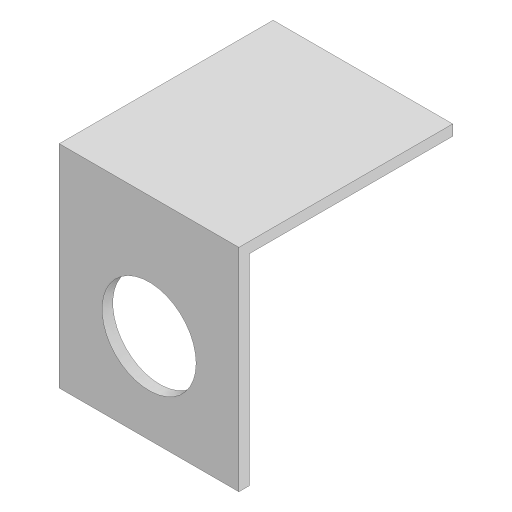
# Autodesk Inventor part: SOPORTE DE NEMA
Saved by Autodesk Inventor 2024 (Build 280153000, 153)
## iProperties
Created: 2024-06-13
Part Number: SOPORTE DE NEMA
Material: Generic
Document SubType Name: Modeling
Designer: Jhuliams
Density: 1 g/cm^3
Appearance: Default
Author: Jhuliams
Autodesk Inventor part; units mm, degrees
ref_plane "YZ Plane" through (0, 0, 0) normal (1, 0, 0) x (0, 1, 0)
ref_plane "XZ Plane" through (0, 0, 0) normal (0, 1, 0) x (-1, 0, 0)
ref_plane "XY Plane" through (0, 0, 0) normal (0, 0, 1) x (1, 0, 0)
sketch "Sketch1" plane through (0, 0, 0) normal (0, 0, 1) x (1, 0, 0)
  line L0 (-21, 21) -> (21, 21)
  line L1 (21, 21) -> (21, -21)
  line L2 (21, -21) -> (-21, -21)
  line L3 (-21, -21) -> (-21, 21)
  line L4 (-21, 21) -> (21, -21) construction
  line L5 (21, 21) -> (-21, -21) construction
  circle A0 centre (0, 0) radius 11
  dimension "d0" = 42
  dimension "d1" = 42
  dimension "d2" = 22
  constraints: 12 end point, 2 midpoint, 2 parallel, 1 centre point, 1 coincident, 1 horizontal, 1 perpendicular
  measures "d0" distance of L1.end L2.end
  measures "d1" distance of L0.end L1.end
  measures "d2" diameter of A0
extrude "Extrusion1" add sketch "Sketch1" along normal blind 2.5
sketch "Sketch2" plane through (-21, 21, 0) normal (0, 1, 0) x (1, 0, 0)
  line L0 (42, 0) -> (0, 0) projected
  line L1 (0, 0) -> (0, -2.5) projected
  line L2 (42, -2.5) -> (0, -2.5) projected
  line L3 (42, 0) -> (42, -2.5) projected
  point P0 (21, 0)
extrude "Extrusion2" add sketch "Sketch2" along normal blind 5
sketch "Sketch3" plane through (0, 0, 2.5) normal (0, 0, 1) x (1, 0, 0)
  line L0 (-21, -21) -> (-21, 26) projected
  line L1 (-21, 26) -> (21, 26)
  line L2 (21, 26) -> (21, 28.5)
  line L3 (21, 28.5) -> (-21, 28.5)
  line L4 (-21, 28.5) -> (-21, 26)
  point P0 (0, 0)
  dimension "d7" = 42
  dimension "d8" = 2.5
  constraints: 8 end point, 2 parallel, 1 horizontal, 1 perpendicular
  measures "d7" distance of L3.end L2.end
  measures "d8" distance of L2.end L1.end
extrude "Extrusion3" add sketch "Sketch3" against normal blind 50
body "Solid1"
